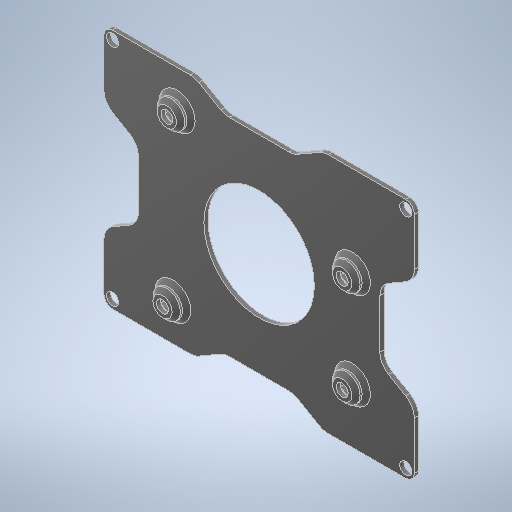
# Autodesk Inventor part: 3D_circuit-fix_arduino
Saved by Autodesk Inventor 2025 (Build 290162000, 162)
## iProperties
Created: 2024-07-24
Part Number: 3D_circuit-fix_arduino
Material: 一般
Document SubType Name: Modeling
Designer: 8326d
Density: 1 g/cm^3
Appearance: 滑らか - 黒
Author: 8326d
## iProperties of the stored document 3D_circuit-fix_arduino_3D プリント.ipt
Created: 2024-08-20
Part Number: 3D_circuit-fix_arduino_3D プリント
Material: 一般
Document SubType Name: Modeling
Designer: 8326d
Density: 1 g/cm^3
Appearance: 既定
Author: 8326d
Autodesk Inventor part; units mm, degrees
ref_plane "YZ Plane" through (0, 0, 0) normal (1, 0, 0) x (0, 1, 0)
ref_plane "XZ Plane" through (0, 0, 0) normal (0, 1, 0) x (-1, 0, 0)
ref_plane "XY Plane" through (0, 0, 0) normal (0, 0, 1) x (1, 0, 0)
sketch "スケッチ1" plane through (0, 0, 0) normal (0, 0, 1) x (1, 0, 0)
  line L0 (-45, -35) -> (45, -35)
  line L1 (45, -35) -> (45, 35)
  line L2 (45, 35) -> (-45, 35)
  line L3 (-45, 35) -> (-45, -35)
  line L4 (-45, -35) -> (45, 35) construction
  line L5 (45, -35) -> (-45, 35) construction
  point P0 (0, 0)
  dimension "d0" = 90
  dimension "d1" = 70
  constraints: 12 end point, 2 midpoint, 2 parallel, 1 horizontal, 1 perpendicular
  measures "d0" distance of L2.end L1.end
  measures "d1" distance of L1.end L0.end
extrude "押し出し1" add sketch "スケッチ1" along normal blind 1.2
sketch "スケッチ2" plane through (0, 0, 1.2) normal (0, 0, 1) x (1, 0, 0)
  line L0 (-42.5, -32.5) -> (42.5, -32.5) construction
  line L1 (42.5, -32.5) -> (42.5, 32.5) construction
  line L2 (42.5, 32.5) -> (-42.5, 32.5) construction
  line L3 (-42.5, 32.5) -> (-42.5, -32.5) construction
  line L4 (-42.5, -32.5) -> (42.5, 32.5) construction
  line L5 (42.5, -32.5) -> (-42.5, 32.5) construction
  point P0 (0, 0)
  dimension "d4" = 85
  dimension "d5" = 65
  constraints: 12 end point, 2 midpoint, 2 parallel, 1 horizontal, 1 perpendicular
  measures "d4" distance of L2.end L1.end
  measures "d5" distance of L1.end L0.end
hole "穴1" at (-42.5, 32.5, 1.2) at (-42.5, -32.5, 1.2) at (42.5, -32.5, 1.2) at (42.5, 32.5, 1.2) direction (0, 0, -1) diameter 3.5 end through all
sketch "スケッチ3" plane through (0, 0, 1.2) normal (0, 0, 1) x (1, 0, 0)
  circle A0 centre (-25, -24.13) radius 4
  circle A1 centre (-23.73, 24.13) radius 4
  circle A2 centre (27.07, 8.89) radius 4
  circle A3 centre (27.07, -19.05) radius 4
  point P0 (0, 0)
  dimension "d13" = 8
  dimension "d14" = 8
  dimension "d15" = 8
  dimension "d16" = 8
  dimension "d17" = 48.26
  dimension "d18" = 1.27
  dimension "d19" = 27.94
  dimension "d20" = 5.08
  dimension "d21" = 52.07
  dimension "d22" = 24.13
  dimension "d23" = 25
  constraints: 4 centre point, 1 vertical alignment
  measures "d13" diameter of A0
  measures "d14" diameter of A1
  measures "d15" diameter of A2
  measures "d16" diameter of A3
  measures "d17" vertical distance of A0.centre A1.centre
  measures "d18" horizontal distance of A0.centre A1.centre
  measures "d19" distance of A3.centre A2.centre
  measures "d20" vertical distance of A3.centre A0.centre
  measures "d21" horizontal distance of A3.centre A0.centre
  measures "d22" vertical distance of A0.centre point (0, 0)
  measures "d23" horizontal distance of A0.centre point (0, 0)
extrude "押し出し2" add sketch "スケッチ3" along normal blind 3
chamfer "面取り1" distance 1.2 angle 45 8 edges at (-29, -24.13, 4.2) (-27.73, 24.13, 4.2) (23.07, 8.89, 4.2) (23.07, -19.05, 4.2) (-27.73, 24.13, 1.2) (-29, -24.13, 1.2) (23.07, 8.89, 1.2) (23.07, -19.05, 1.2)
sketch "スケッチ4" plane through (-25, -24.13, 4.2) normal (0, 0, 1) x (1, 0, 0)
  circle A0 centre (1.27, 48.26) radius 2.8 projected
  circle A1 centre (0, 0) radius 2.8 projected
  circle A2 centre (52.07, 5.08) radius 2.8 projected
  circle A3 centre (52.07, 33.02) radius 2.8 projected
  point P0 (25, 24.13)
hole "穴2" at (-23.73, 24.13, 4.2) at (-25, -24.13, 4.2) at (27.07, -19.05, 4.2) at (27.07, 8.89, 4.2) direction (0, 0, -1) diameter 3.5 end through all
sketch "スケッチ5" plane through (0, 0, 0) normal (0, 0, -1) x (-1, 0, 0)
  circle A0 centre (25, -24.13) radius 1.75 projected
  circle A1 centre (23.73, 24.13) radius 1.75 projected
  circle A2 centre (-27.07, 8.89) radius 1.75 projected
  circle A3 centre (-27.07, -19.05) radius 1.75 projected
  line L0 (25, -27.3632) -> (22.2, -25.7466)
  line L1 (22.2, -25.7466) -> (22.2, -22.5134)
  line L2 (22.2, -22.5134) -> (25, -20.8968)
  line L3 (25, -20.8968) -> (27.8, -22.5134)
  line L4 (27.8, -22.5134) -> (27.8, -25.7466)
  line L5 (27.8, -25.7466) -> (25, -27.3632)
  line L6 (23.73, 20.8968) -> (20.93, 22.5134)
  line L7 (20.93, 22.5134) -> (20.93, 25.7466)
  line L8 (20.93, 25.7466) -> (23.73, 27.3632)
  line L9 (23.73, 27.3632) -> (26.53, 25.7466)
  line L10 (26.53, 25.7466) -> (26.53, 22.5134)
  line L11 (26.53, 22.5134) -> (23.73, 20.8968)
  circle A4 centre (-27.07, -19.05) radius 2.8 projected
  line L12 (-27.07, -22.2832) -> (-29.87, -20.6666)
  line L13 (-29.87, -20.6666) -> (-29.87, -17.4334)
  line L14 (-29.87, -17.4334) -> (-27.07, -15.8168)
  line L15 (-27.07, -15.8168) -> (-24.27, -17.4334)
  line L16 (-24.27, -17.4334) -> (-24.27, -20.6666)
  line L17 (-24.27, -20.6666) -> (-27.07, -22.2832)
  line L18 (-27.07, 5.6568) -> (-29.87, 7.2734)
  line L19 (-29.87, 7.2734) -> (-29.87, 10.5066)
  line L20 (-29.87, 10.5066) -> (-27.07, 12.1232)
  line L21 (-27.07, 12.1232) -> (-24.27, 10.5066)
  line L22 (-24.27, 10.5066) -> (-24.27, 7.2734)
  line L23 (-24.27, 7.2734) -> (-27.07, 5.6568)
  point P0 (0, 0)
  dimension "d36" = 5.6
  dimension "d37" = 5.6
  dimension "d38" = 5.6
  dimension "d39" = 5.6
  constraints: 48 end point, 4 coincident, 4 vertical alignment, 52 other
  measures "d36" distance between parallel lines of L3 L0
  measures "d37" distance between parallel lines of L9 L6
  measures "d38" distance between parallel lines of L12 L15
  measures "d39" distance between parallel lines of L21 L18
extrude "押し出し3" cut sketch "スケッチ5" against normal blind 3 contours A2 | A3 | L0 L1 L2 L3 L4 L5 | L6 L7 L8 L9 L10 L11 | A4 | L16 L17 A4 | A4 L15 L16 | A4 L14 L15 | L17 L12 A4 | A4 L13 L14 | L12 L13 A4 | L18 L19 L20 L21 L22 L23
sketch "スケッチ6" plane through (0, 0, 3) normal (0, 0, -1) x (-1, 0, 0)
  line L0 (27.8, -22.5134) -> (27.8, -25.7466) projected
  line L1 (25, -20.8968) -> (27.8, -22.5134) projected
  line L2 (22.2, -22.5134) -> (25, -20.8968) projected
  line L3 (22.2, -25.7466) -> (22.2, -22.5134) projected
  line L4 (25, -27.3632) -> (22.2, -25.7466) projected
  line L5 (27.8, -25.7466) -> (25, -27.3632) projected
  circle A0 centre (25, -24.13) radius 1.75 projected
  line L6 (26.53, 25.7466) -> (26.53, 22.5134) projected
  line L7 (23.73, 27.3632) -> (26.53, 25.7466) projected
  line L8 (20.93, 25.7466) -> (23.73, 27.3632) projected
  line L9 (20.93, 22.5134) -> (20.93, 25.7466) projected
  line L10 (23.73, 20.8968) -> (20.93, 22.5134) projected
  line L11 (26.53, 22.5134) -> (23.73, 20.8968) projected
  circle A1 centre (23.73, 24.13) radius 1.75 projected
  circle A2 centre (-27.07, 8.89) radius 1.75 projected
  line L12 (-24.27, 10.5066) -> (-24.27, 7.2734) projected
  line L13 (-27.07, 12.1232) -> (-24.27, 10.5066) projected
  line L14 (-29.87, 10.5066) -> (-27.07, 12.1232) projected
  line L15 (-29.87, 7.2734) -> (-29.87, 10.5066) projected
  line L16 (-27.07, 5.6568) -> (-29.87, 7.2734) projected
  line L17 (-24.27, 7.2734) -> (-27.07, 5.6568) projected
  circle A3 centre (-27.07, -19.05) radius 1.75 projected
  line L18 (-29.87, -20.6666) -> (-29.87, -17.4334) projected
  line L19 (-27.07, -22.2832) -> (-29.87, -20.6666) projected
  line L20 (-24.27, -20.6666) -> (-27.07, -22.2832) projected
  line L21 (-24.27, -17.4334) -> (-24.27, -20.6666) projected
  line L22 (-27.07, -15.8168) -> (-24.27, -17.4334) projected
  line L23 (-29.87, -17.4334) -> (-27.07, -15.8168) projected
  line L24 (27.8, -22.5134) -> (27.8, -25.7466) projected
  line L25 (27.8, -24.5341) -> (23.95, -26.7569)
  line L26 (23.25, -26.3528) -> (23.25, -21.9072)
  line L27 (23.95, -21.5031) -> (27.8, -23.7259)
  line L28 (27.8, -25.7466) -> (25, -27.3632) projected
  line L29 (25, -20.8968) -> (27.8, -22.5134) projected
  circle A4 centre (25, -24.13) radius 1.75 projected
  line L30 (20.93, 25.7466) -> (23.73, 27.3632) projected
  line L31 (21.98, 26.3528) -> (21.98, 21.9072)
  line L32 (22.68, 21.5031) -> (26.53, 23.7259)
  line L33 (26.53, 25.7466) -> (26.53, 22.5134) projected
  line L34 (26.53, 24.5341) -> (22.68, 26.7569)
  line L35 (26.53, 22.5134) -> (23.73, 20.8968) projected
  line L36 (23.73, 27.3632) -> (26.53, 25.7466) projected
  circle A5 centre (23.73, 24.13) radius 1.75 projected
  line L37 (-28.82, 6.6672) -> (-28.82, 11.1128)
  line L38 (-28.12, 11.5169) -> (-24.27, 9.2941)
  line L39 (-24.27, 10.5066) -> (-24.27, 7.2734) projected
  line L40 (-24.27, 8.4859) -> (-28.12, 6.2631)
  line L41 (-27.07, 12.1232) -> (-24.27, 10.5066) projected
  line L42 (-24.27, 7.2734) -> (-27.07, 5.6568) projected
  circle A6 centre (-27.07, 8.89) radius 1.75 projected
  line L43 (-24.27, -19.4541) -> (-28.12, -21.6769)
  line L44 (-28.82, -21.2728) -> (-28.82, -16.8272)
  line L45 (-28.12, -16.4231) -> (-24.27, -18.6459)
  line L46 (-24.27, -20.6666) -> (-27.07, -22.2832) projected
  line L47 (-27.07, -15.8168) -> (-24.27, -17.4334) projected
  circle A7 centre (-27.07, -19.05) radius 1.75 projected
  point P0 (0, 0)
  point P1 (-24.27, 8.4859)
  point P2 (26.53, 23.7259)
  point P3 (27.8, -24.5341)
  constraints: 24 end point, 24 point on line, 12 tangent, 8 parallel, 4 vertical
extrude "押し出し4" add sketch "スケッチ6" along normal blind 0.2 contours L0 L27 L2 L1 | L0 L5 L4 L25 | L26 L4 L3 L2 | L6 L34 L8 L7 | L6 L11 L10 L32 | L31 L10 L9 L8 | L38 L14 L13 L12 | L40 L12 L17 L16 | L37 L16 L15 L14 | L45 L23 L22 L21 | L43 L21 L20 L19 | L44 L19 L18 L23
fillet "フィレット1" radius 2.5 4 edges at (-45, -35, 0.6) (-45, 35, 0.6) (45, -35, 0.6) (45, 35, 0.6)
sketch "スケッチ7" plane through (0, 0, 1.2) normal (0, 0, 1) x (1, 0, 0)
  line L0 (42.5, 35) -> (-42.5, 35) projected
  line L1 (-10, 35) -> (10, 35)
  line L2 (10, 35) -> (10, 30)
  line L3 (10, 30) -> (-10, 30)
  line L4 (-10, 30) -> (-10, 35)
  line L5 (-10, 30) -> (-18.6603, 35)
  line L6 (10, 30) -> (18.6603, 35)
  line L7 (45, -32.5) -> (45, 32.5) projected
  line L8 (45, 10) -> (35, 10)
  line L9 (35, 10) -> (35, -10)
  line L10 (35, -10) -> (45, -10)
  line L11 (45, -10) -> (45, 10)
  line L12 (35, 10) -> (45, 15.7735)
  line L13 (45, 0) -> (35, 0)
  point P0 (0, 0)
  point P1 (0, 35)
  dimension "d45" = 20
  dimension "d46" = 5
  dimension "d47" = 30
  dimension "d48" = 30
  dimension "d52" = 20
  dimension "d53" = 10
  constraints: 24 end point, 5 midpoint, 5 parallel, 5 point on line, 2 horizontal, 2 perpendicular
  measures "d45" distance of L2.end L3.end
  measures "d46" distance of L1.end L2.end
  measures "d47" angle of L0 L6
  measures "d48" angle of L0 L5
  measures "d52" distance of L8.end L9.end
  measures "d53" distance of L8.start L8.end
extrude "押し出し5" cut sketch "スケッチ7" against normal through all contours L6 L2 L0 | L2 L3 L4 L0 | L4 L5 L0 | L13 L9 L8 L7 | L8 L12 L7
mirror "ミラー1" about plane through (0, 0, 0) normal (0, 1, 0) of "押し出し5"
mirror "ミラー2" about plane through (0, 0, 0) normal (1, 0, 0) of "押し出し5", "ミラー1"
fillet "フィレット2" radius 5 16 edges at (-18.6603, -35, 0.6) (-10, -30, 0.6) (10, -30, 0.6) (18.6603, -35, 0.6) (10, 30, 0.6) (-10, 30, 0.6) (-18.6603, 35, 0.6) (18.6603, 35, 0.6) (-45, -15.7735, 0.6) (-35, -10, 0.6) (-35, 10, 0.6) (-45, 15.7735, 0.6) (45, -15.7735, 0.6) (35, -10, 0.6) (35, 10, 0.6) (45, 15.7735, 0.6)
sketch "スケッチ8" plane through (0, 0, 1.2) normal (0, 0, 1) x (1, 0, 0)
  circle A0 centre (0, 0) radius 16
  dimension "d54" = 32
  constraints: 1 centre point, 1 coincident
  measures "d54" diameter of A0
extrude "押し出し6" cut sketch "スケッチ8" against normal through all
equation "\"d22\" = 0.5 * d17"
equation "\"d37\" = d36"
equation "\"d38\" = d36"
equation "\"d39\" = d36"
equation "\"d48\" = d47"
